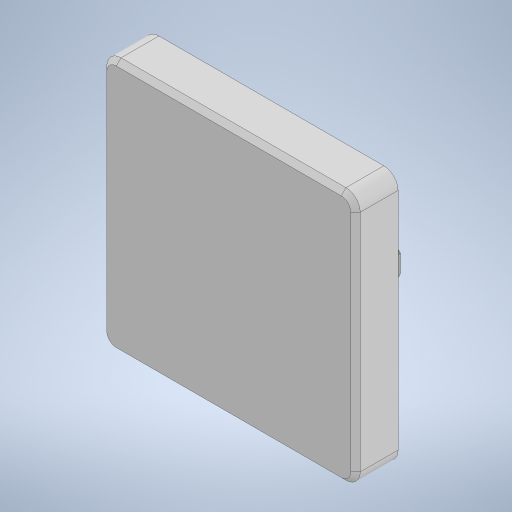
# Autodesk Inventor part: horni_vlozka
Saved by Autodesk Inventor 2024 (Build 280153000, 153)
## iProperties
Created: 2024-03-13
Part Number: horni_vlozka
Material: Všeobecné
Document SubType Name: Modeling
Designer: 42060
Density: 1 g/cm^3
Appearance: Výchozí
Author: 42060
Autodesk Inventor part; units mm, degrees
ref_plane "YZ Plane" through (0, 0, 0) normal (1, 0, 0) x (0, 1, 0)
ref_plane "XZ Plane" through (0, 0, 0) normal (0, 1, 0) x (-1, 0, 0)
ref_plane "XY Plane" through (0, 0, 0) normal (0, 0, 1) x (1, 0, 0)
sketch "Náčrt1" plane through (0, 0, 0) normal (0, 1, 0) x (-1, 0, 0)
  line L0 (49.5, 49.5) -> (-49.5, 49.5)
  line L1 (-49.5, 49.5) -> (-49.5, -49.5)
  line L2 (-49.5, -49.5) -> (49.5, -49.5)
  line L3 (49.5, -49.5) -> (49.5, 49.5)
  line L4 (49.5, 49.5) -> (-49.5, -49.5) construction
  line L5 (-49.5, 49.5) -> (49.5, -49.5) construction
  line L6 (53.5, 53.5) -> (-53.5, 53.5)
  line L7 (-53.5, 53.5) -> (-53.5, -53.5)
  line L8 (-53.5, -53.5) -> (53.5, -53.5)
  line L9 (53.5, -53.5) -> (53.5, 53.5)
  line L10 (53.5, 53.5) -> (-53.5, -53.5) construction
  line L11 (-53.5, 53.5) -> (53.5, -53.5) construction
  point P0 (0, 0)
  dimension "d1" = 99
  dimension "d2" = 4
  constraints: 24 end point, 4 midpoint, 4 parallel, 4 perpendicular, 2 horizontal
  measures "d1" distance of L0.end L1.end
  measures "d2" distance between parallel lines of L1 L7
extrude "Vysunutí1" add sketch "Náčrt1" along normal blind 2 contours L3 L2 L1 L0
extrude "Vysunutí2" add sketch "Náčrt1" along normal blind 18
fillet "Zaoblení1" radius 6 4 edges at (53.5, 9, 53.5) (53.5, 9, -53.5) (-53.5, 9, -53.5) (-53.5, 9, 53.5)
chamfer "Zkosení1" distance 2 angle 45 8 edges at (0, 0, 53.5) (51.7426, 0, 51.7426) (53.5, 0, 0) (51.7426, 0, -51.7426) (0, 0, -53.5) (-51.7426, 0, -51.7426) (-53.5, 0, 0) (-51.7426, 0, 51.7426)
sketch "Náčrt2" plane through (0, 2, 0) normal (0, 1, 0) x (1, 0, 0)
  line L0 (47.25, -18.75) -> (23, -43)
  line L1 (23, -43) -> (-23, -43)
  line L2 (-23, -43) -> (-47.25, -18.75)
  line L3 (-49.75, -19.7855) -> (-24.0355, -45.5)
  line L4 (-24.0355, -45.5) -> (24.0355, -45.5)
  line L5 (24.0355, -45.5) -> (49.75, -19.7855)
  line L6 (49.75, -19.7855) -> (49.75, -7.5)
  line L7 (49.75, -7.5) -> (47.25, -7.5)
  line L8 (47.25, -7.5) -> (47.25, -18.75)
  line L9 (-47.25, -18.75) -> (-47.25, -7.5)
  line L10 (-47.25, -7.5) -> (-49.75, -7.5)
  line L11 (-49.75, -7.5) -> (-49.75, -19.7855)
  line L12 (49.5, -49.5) -> (-49.5, -49.5) projected
  line L13 (49.5, 49.5) -> (49.5, -49.5) projected
  point P0 (0, 0)
  point P1 (0, -45.5)
  point P2 (0, -49.5)
  point P3 (49.5, -20.0355)
  point P4 (49.5, -7.5)
  dimension "d12" = 2.5
  dimension "d13" = 2.5
  dimension "d14" = 2.5
  dimension "d15" = 46
  dimension "d16" = 135
  dimension "d17" = 2.5
  dimension "d18" = 2.5
  dimension "d19" = 38
  dimension "d20" = 99.5
  dimension "d21" = 11.25
  dimension "d22" = 4
  constraints: 24 end point, 4 perpendicular, 3 parallel, 2 midpoint, 2 vertical, 1 horizontal, 1 horizontal alignment, 1 vertical alignment
  measures "d12" distance between parallel lines of L4 L1
  measures "d13" distance between parallel lines of L3 L2
  measures "d14" distance between parallel lines of L5 L0
  measures "d15" distance of L0.end L1.end
  measures "d16" angle of L1 L0
  measures "d17" distance between parallel lines of L11 L9
  measures "d18" distance between parallel lines of L6 L8
  measures "d19" distance between parallel lines of L7 L4
  measures "d20" distance between parallel lines of L11 L6
  measures "d21" distance of L7.end L0.start
  measures "d22" distance between parallel lines of L4 L12
extrude "Vysunutí3" add sketch "Náčrt2" along normal blind 21 contours L8 L7 L13 L5 L4 L3 L11 L10 L9 L2 L1 L0
sketch "Náčrt3" plane through (0, 2, 0) normal (0, 1, 0) x (1, 0, 0)
  circle A0 centre (-8, 43.25) radius 2.5
  circle A1 centre (-8, 43.25) radius 1.5
  line L0 (49.5, 49.5) -> (49.5, -7.5) projected
  line L1 (-49.5, -7.5) -> (-49.5, 49.5) projected
  line L2 (-49.5, 49.5) -> (49.5, 49.5) projected
  point P0 (0, 0)
  dimension "d27" = 3
  dimension "d28" = 5
  dimension "d39" = 41.5
  dimension "d43" = 6.25
  constraints: 2 centre point, 1 coincident
  measures "d27" diameter of A1
  measures "d28" diameter of A0
  measures "d39" distance from line of L1 A0.centre
  measures "d43" distance from line of L2 A0.centre
extrude "Vysunutí4" add sketch "Náčrt3" along normal blind 18 contours A1
extrude "Vysunutí5" add sketch "Náčrt3" along normal blind 17
chamfer "Zkosení2" distance 1 angle 45 1 edges at (-9.5, 19, -43.25)
chamfer "Zkosení3" distance 2 angle 45 11 edges at (-10.5, 2, -43.25) (-35.125, 2, 30.875) (-47.25, 2, 13.125) (0, 2, 43) (35.125, 2, 30.875) (47.25, 2, 13.125) (48.375, 2, 7.5) (-48.375, 2, 7.5) (36.7678, 2, 32.7678) (0, 2, 45.5) (-36.7678, 2, 32.7678)
chamfer "Zkosení4" distance 5 angle 45 2 edges at (-48.5, 23, 7.5) (48.375, 23, 7.5)
